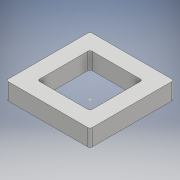
# Autodesk Inventor part: Ram(Nästankvadratisk
Saved by Autodesk Inventor 2018 (Build 220112000, 112)
## iProperties
Created: 2018-02-08
Part Number: Ram(Nästankvadratisk
Material: Generic
Document SubType Name: Modeling
Designer: davton
Density: 1 g/cm^3
Appearance: Default
Author: davton
Autodesk Inventor part; units mm, degrees
ref_plane "YZ Plane" through (0, 0, 0) normal (1, 0, 0) x (0, 1, 0)
ref_plane "XZ Plane" through (0, 0, 0) normal (0, 1, 0) x (-1, 0, 0)
ref_plane "XY Plane" through (0, 0, 0) normal (0, 0, 1) x (1, 0, 0)
sketch "Sketch1" plane through (0, 0, 0) normal (0, 0, 1) x (1, 0, 0)
  point P0 (0, 0)
sketch "Sketch2" plane through (0, 0, 0) normal (0, 0, 1) x (1, 0, 0)
  line L0 (-22.3056, -24.3056) -> (22.3056, -24.3056)
  line L1 (24.3056, -22.3056) -> (24.3056, 22.3056)
  line L2 (22.3056, 24.3056) -> (-22.3056, 24.3056)
  line L3 (-24.3056, 22.3056) -> (-24.3056, -22.3056)
  line L4 (-24.3056, -24.3056) -> (24.3056, 24.3056) construction
  line L5 (24.3056, -24.3056) -> (-24.3056, 24.3056) construction
  line L6 (-36.8889, -38.8889) -> (36.8889, -38.8889)
  line L7 (38.8889, -36.8889) -> (38.8889, 36.8889)
  line L8 (36.8889, 38.8889) -> (-36.8889, 38.8889)
  line L9 (-38.8889, 36.8889) -> (-38.8889, -36.8889)
  line L10 (-38.8889, -38.8889) -> (38.8889, 38.8889) construction
  line L11 (38.8889, -38.8889) -> (-38.8889, 38.8889) construction
  arc A0 (-36.8889, 38.8889) -> (-38.8889, 36.8889) centre (-36.8889, 36.8889) ccw
  arc A1 (38.8889, 36.8889) -> (36.8889, 38.8889) centre (36.8889, 36.8889) ccw
  arc A2 (36.8889, -38.8889) -> (38.8889, -36.8889) centre (36.8889, -36.8889) ccw
  arc A3 (-38.8889, -36.8889) -> (-36.8889, -38.8889) centre (-36.8889, -36.8889) ccw
  arc A4 (-24.3056, -22.3056) -> (-22.3056, -24.3056) centre (-22.3056, -22.3056) ccw
  arc A5 (22.3056, -24.3056) -> (24.3056, -22.3056) centre (22.3056, -22.3056) ccw
  arc A6 (24.3056, 22.3056) -> (22.3056, 24.3056) centre (22.3056, 22.3056) ccw
  arc A7 (-22.3056, 24.3056) -> (-24.3056, 22.3056) centre (-22.3056, 22.3056) ccw
  point P0 (0, 0)
  dimension "HL" = 48.6111
  dimension "d1" = 24.3056
  dimension "d2" = 77.7778
  dimension "d3" = 38.8889
  dimension "d4" = 2
  constraints: 24 end point, 16 point on circle, 16 point on line, 16 tangent, 8 centre point, 7 equal radius, 4 midpoint, 4 parallel, 2 horizontal, 2 perpendicular
  measures "HL" distance of L5.end L4.end
  measures "d1" distance from line of L2 point (0, 0)
  measures "d2" distance of L11.end L10.end
  measures "d3" distance from line of L8 point (0, 0)
  measures "d4" radius of A0
extrude "Extrusion1" add sketch "Sketch2" along normal blind 15.5556
equation "\"d1\" = 0.5 * HL"
equation "\"d2\" = 1.6 * HL"
equation "\"d3\" = 0.8 * HL"
equation "\"d5\" = 0.32 * HL"
body "Solid1"
